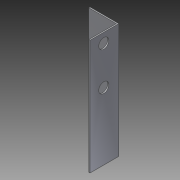
# Autodesk Inventor part: Shooter Main Gear Guide Bar
Saved by Autodesk Inventor 2014 SP1 (Build 180222100, 222)
## iProperties
Created: 2013-12-13
Part Number: Shooter Main Gear Guide Bar
Material: Aluminum 6061
Document SubType Name: Modeling
Designer: Moses
Density: 2.71 g/cm^3
Appearance: Aluminum - Flat
Mass: 5.96066 g
Surface Area: 57.5595 cm^2
Volume: 2.19951 cm^3
Author: Moses
Autodesk Inventor part; units mm, degrees
ref_plane "YZ Plane" through (0, 0, 0) normal (1, 0, 0) x (0, 1, 0)
ref_plane "XZ Plane" through (0, 0, 0) normal (0, 1, 0) x (-1, 0, 0)
ref_plane "XY Plane" through (0, 0, 0) normal (0, 0, 1) x (1, 0, 0)
sketch "Sketch1" plane through (0, 0, 0) normal (0, 1, 0) x (-1, 0, 0)
  line L0 (0, 0) -> (0, 19.05)
  line L1 (0, 19.05) -> (0.7937, 19.05)
  line L2 (0.7937, 19.05) -> (0.7938, 0.7937)
  line L3 (0.7938, 0.7937) -> (19.05, 0.7937)
  line L4 (19.05, 0.7937) -> (19.05, 0)
  line L5 (19.05, 0) -> (0, 0)
  dimension "d0" = 19.05
  dimension "d1" = 0.7937
  constraints: 12 end point, 3 horizontal, 3 vertical, 2 perpendicular
  measures "d0" distance of L0.start L0.end
  measures "d1" distance of L0.end L1.end
extrude "Extrusion1" add sketch "Sketch1" along normal blind 76.2
sketch "Sketch2" plane through (0, 0, 19.05) normal (1, 0, 0) x (0, 0, -1)
  circle A0 centre (9.1281, 69.85) radius 3.3782
  circle A1 centre (9.1281, 44.45) radius 3.3782
  line L0 (0, 76.2) -> (19.05, 76.2) projected
  line L1 (0, 0) -> (0, 76.2) projected
  line L2 (18.2563, 0) -> (18.2563, 76.2) projected
  line L3 (18.2563, 38.1) -> (0, 38.1) construction
  line L4 (9.1281, 38.1) -> (9.1281, 76.2) construction
  dimension "d5" = 6.7564
  dimension "d18" = 25.4
  dimension "d19" = 6.35
  constraints: 4 end point, 3 midpoint, 3 point on line, 2 centre point, 1 equal radius, 1 vertical
  measures "d5" diameter of A0
  measures "d18" distance of A1.centre A0.centre
  measures "d19" distance of A0.centre L4.end
extrude "Extrusion2" cut sketch "Sketch2" against normal through all
body "Solid1"
